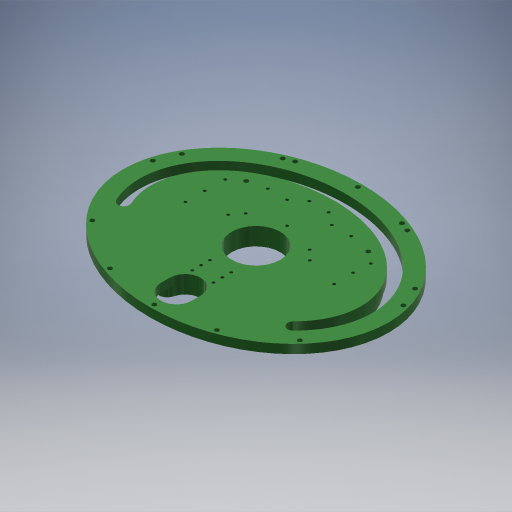
# Autodesk Inventor part: 24_0497_006
Saved by Autodesk Inventor 2024.3 (Build 283343000, 343)
## iProperties
Created: 2024-05-28
Part Number: 24_0497_006
Material: LCP-Kunststoff
Document SubType Name: Modeling
Designer: Vogel
Density: 1.626 g/cm^3
Appearance: Glatt - Waldgrün
Author: Vogel
Autodesk Inventor part; units mm, degrees
ref_plane "YZ Plane" through (0, 0, 0) normal (1, 0, 0) x (0, 1, 0)
ref_plane "XZ Plane" through (0, 0, 0) normal (0, 1, 0) x (-1, 0, 0)
ref_plane "XY Plane" through (0, 0, 0) normal (0, 0, 1) x (1, 0, 0)
sketch "Skizze1" plane through (0, 0, 0) normal (0, 0, 1) x (1, 0, 0)
  line L0 (-210, 0) -> (210, 0) projected
  line L1 (0, -168) -> (0, 168) projected
  ellipse E0 centre (0, 0) end of major axis (-150, 0) minor radius 120
  line L2 (0, 120) -> (0, -120) construction
  line L3 (-150, 0) -> (150, 0) construction
  dimension "d0" = 300
  dimension "d1" = 240
  constraints: 4 end point, 4 point on line, 1 coincident, 6 other
  measures "d0" distance of L3.start L3.end
  measures "d1" distance of L2.start L2.end
extrude "Extrusion1" add sketch "Skizze1" along normal blind 10
sketch "Skizze2" plane through (0, 0, 10) normal (0, 0, 1) x (1, 0, 0)
  ellipse E0 centre (0, 0) end of major axis (-150, 0) minor radius 120 projected
  line L0 (0, -168) -> (0, 168) projected
  line L1 (-210, 0) -> (210, 0) projected
  line L2 (-131.5, 0) -> (131.5, 0)
  line L3 (0, 101.5) -> (0, -101.5)
  ellipse E1 centre (0, 0) end of major axis (-131.5, 0) minor radius 101.5
  line L4 (0, 0) -> (-124.2275, -33.2867) construction
  line L5 (0, 0) -> (105.3012, -60.7957) construction
  ellipse E2 centre (0, 0) end of major axis (118.5, 0) minor radius 88.5
  line L6 (0, 0) -> (80.349, 80.349) construction
  line L7 (80.349, 80.349) -> (73.764, 69.2632)
  line L8 (67.3414, 73.0783) -> (84.3123, 62.9974)
  arc A0 (94.9826, -52.9176) -> (105.1165, -60.6891) centre (99.5391, -57.469) ccw
  arc A1 (-124.1391, -33.263) -> (-112.0157, -28.8739) centre (-117.8892, -31.5883) ccw
  point P0 (0, 120)
  point P1 (150, 0)
  point P2 (-150, 0)
  point P3 (0, -120)
  point P4 (118.5, 0)
  point P5 (-96, 0)
  point P6 (0, 88.5)
  point P7 (-123.7552, -34.3188)
  point P8 (104.0928, -62.0231)
  dimension "d7" = 18.5
  dimension "d8" = 18.5
  dimension "d9" = 31.5
  dimension "d10" = 31.5
  dimension "d11" = 45
  dimension "d12" = 90
  dimension "d13" = 12.8941
  dimension "d14" = 30
  dimension "d15" = 15
  constraints: 16 point on line, 14 end point, 7 coincident, 4 point on circle, 2 centre point, 2 horizontal, 2 symmetric about line, 24 other
  measures "d7" distance of point (0, 120) L3.start
  measures "d8" distance of L2.end point (150, 0)
  measures "d9" distance of point (0, 120) point (0, 88.5)
  measures "d10" distance of point (150, 0) point (118.5, 0)
  measures "d11" angle of L6 L1
  measures "d12" angle of L8 L7
  measures "d13" distance of L6.end L7.end
  measures "d14" angle of L2 L5
  measures "d15" angle of L2 L4
extrude "Extrusion2" cut sketch "Skizze2" against normal through all contours E1 L0 E2 L1 | L1 E2 A1 E1 | E1 L7 E2 L0 | E1 A0 E2 L1 | L1 E2 L7 E1
sketch "Skizze3" plane through (0, 0, 0) normal (0, 0, -1) x (-1, 0, 0)
  arc A0 (-104.0928, -62.0231) -> (-94.9826, -52.9176) centre (-99.5391, -57.469) ccw projected
  ellipse E0 centre (0, 0) end of major axis (131.5, 0) minor radius 101.5 (123.7552, -34.3188) -> (-104.0928, -62.0231) ccw projected
  arc A1 (112.0157, -28.8739) -> (123.7552, -34.3188) centre (117.8892, -31.5883) ccw projected
  ellipse E1 centre (0, 0) end of major axis (118.5, 0) minor radius 88.5 (112.0157, -28.8739) -> (-94.9826, -52.9176) ccw projected
  ellipse E2 centre (0, 0) end of major axis (150, 0) minor radius 120 projected
  line L0 (0, 0) -> (0, 120)
  line L1 (0, 0) -> (-150, 0)
  ellipse E3 centre (0, 0) end of major axis (-116, 0) minor radius 86
  circle A2 centre (0, -95.478) radius 8.75 projected
  line L2 (210, 0) -> (-210, 0) projected
  line L3 (0, -168) -> (0, 168) projected
  point P0 (0, 86)
  point P1 (-116, 0)
  point P2 (0, -86)
  point P3 (0, -86.728)
  dimension "d18" = 34
  dimension "d19" = 34
  constraints: 4 end point, 3 point on line, 2 horizontal, 1 coincident, 1 vertical, 1 vertical alignment, 11 other
  measures "d18" distance of point (-116, 0) L1.end
  measures "d19" distance of point (0, 86) L0.end
extrude "Extrusion3" add sketch "Skizze3" along normal blind 10 contours E3 L0 L1 | L1 L3 E3 | E3 L2 L0 | L2 E3 L3
sketch "Skizze4" plane through (0, 0, 10) normal (0, 0, 1) x (1, 0, 0)
  line L0 (-210, 0) -> (210, 0) projected
  line L1 (0, -168) -> (0, 168) projected
  circle A0 centre (0, -80) radius 17.5
  point P0 (0, 0)
  dimension "d22" = 35
  dimension "d23" = 80
  constraints: 1 centre point, 1 point on line
  measures "d22" diameter of A0
  measures "d23" distance from line of A0.centre L0
extrude "Extrusion4" cut sketch "Skizze4" against normal through all
sketch "Skizze5" plane through (0, 0, 10) normal (0, 0, 1) x (1, 0, 0)
  circle A0 centre (0, 0) radius 27.5
  dimension "d26" = 55
  constraints: 1 centre point, 1 coincident
  measures "d26" diameter of A0
extrude "Extrusion5" cut sketch "Skizze5" against normal through all
sketch "Skizze6" plane through (0, 0, -10) normal (0, 0, -1) x (-1, 0, 0)
  line L0 (210, 0) -> (-210, 0) projected
  line L1 (0, -168) -> (0, 168) projected
  line L2 (-12, -50) -> (-12, -40)
  line L3 (12, -50) -> (12, -40)
  line L4 (12, -50) -> (12, -60)
  line L5 (-12, -50) -> (-12, -60)
  point P0 (0, 0)
  point P1 (12, -45)
  dimension "d29" = 24
  dimension "d30" = 50
  dimension "d31" = 10
  dimension "d89" = 10
  constraints: 8 end point, 6 coincident, 4 vertical, 3 horizontal alignment, 1 midpoint, 1 other
  measures "d29" distance from line of L2 point (12, -45)
  measures "d30" distance from line of L0 L3.start
  measures "d31" distance of L3.end L3.start
  measures "d89" distance of L4.start L4.end
hole "Bohrung1" at (12, -50, -10) at (12, -40, -10) at (-12, -40, -10) at (-12, -50, -10) at (-12, -60, -10) at (12, -60, -10) direction (0, 0, 1) diameter 3.242 end through all thread size "M4x0.7" class "6H" standard "ISO Metric profile"
sketch "Skizze7" plane through (0, 0, 0) normal (0, 0, -1) x (-1, 0, 0)
  circle A0 centre (0, -115) radius 1.621 projected
  circle A1 centre (-117.2282, -67.6817) radius 1.621 projected
  circle A2 centre (117.2282, -67.6817) radius 1.621 projected
  circle A3 centre (0, 115) radius 1.621 projected
  circle A4 centre (131.7852, 47.9659) radius 1.621 projected
  circle A5 centre (70.3971, 100.5374) radius 1.621 projected
  circle A6 centre (-70.3971, 100.5374) radius 1.621 projected
  circle A7 centre (-131.7852, 47.9659) radius 1.621 projected
  arc A8 (16.8617, 59.8458) -> (2.0406, 61.4653) centre (0.7319, -19.1414) ccw projected
  arc A9 (18.3431, 57.2081) -> (16.8617, 59.8458) centre (16.4616, 57.8862) ccw projected
  line L0 (18.3431, 57.2081) -> (11.1831, 37.3438) projected
  arc A10 (8.9188, 36.0589) -> (11.1831, 37.3438) centre (9.3016, 38.0219) ccw projected
  arc A11 (8.9188, 36.0589) -> (-6.3449, 36.18) centre (0.9627, -4.7433) ccw projected
  arc A12 (-8.5965, 37.5246) -> (-6.3449, 36.18) centre (-6.6965, 38.1489) ccw projected
  line L1 (-8.5965, 37.5246) -> (-15.1484, 57.464) projected
  arc A13 (-13.6228, 60.053) -> (-15.1484, 57.464) centre (-13.2484, 58.0883) ccw projected
  arc A14 (2.0406, 61.4653) -> (-13.6228, 60.053) centre (1.3614, -18.5666) ccw projected
  line L2 (6.9792, -31.0574) -> (-7.1206, -31.0613) projected
  arc A15 (-9.1211, -29.0618) -> (-7.1206, -31.0613) centre (-7.1211, -29.0613) ccw projected
  line L3 (-9.1211, -29.0618) -> (-9.1234, -20.9579) projected
  arc A16 (-7.1239, -18.9573) -> (-9.1234, -20.9579) centre (-7.1234, -20.9573) ccw projected
  line L4 (-7.1239, -18.9573) -> (6.9759, -18.9534) projected
  arc A17 (8.9764, -20.9528) -> (6.9759, -18.9534) centre (6.9764, -20.9534) ccw projected
  line L5 (8.9764, -20.9528) -> (8.9787, -29.0568) projected
  arc A18 (6.9792, -31.0574) -> (8.9787, -29.0568) centre (6.9787, -29.0574) ccw projected
  line L6 (56.8804, 38.6385) -> (35.5944, 25.5797) projected
  arc A19 (33.209, 25.7992) -> (35.5944, 25.5797) centre (34.5485, 27.2844) ccw projected
  arc A20 (33.209, 25.7992) -> (21.3418, 32.6941) centre (10.9014, 1.0642) ccw projected
  arc A21 (20.1931, 35.5138) -> (21.3418, 32.6941) centre (21.9687, 34.5933) ccw projected
  line L7 (20.1931, 35.5138) -> (30.1934, 54.8027) projected
  arc A22 (32.5335, 55.8009) -> (30.1934, 54.8027) centre (31.9689, 53.8822) ccw projected
  arc A23 (57.1918, 41.8123) -> (32.5335, 55.8009) centre (14.9685, -3.8891) ccw projected
  arc A24 (56.8804, 38.6385) -> (57.1918, 41.8123) centre (55.8346, 40.3433) ccw projected
  line L8 (-27.611, 55.4356) -> (-18.0818, 35.9123) projected
  arc A25 (-19.301, 33.1204) -> (-18.0818, 35.9123) centre (-19.8791, 35.035) ccw projected
  arc A26 (-19.301, 33.1204) -> (-31.3271, 26.5166) centre (-9.7404, 1.4574) ccw projected
  arc A27 (-33.7193, 26.353) -> (-31.3271, 26.5166) centre (-32.6324, 28.0319) ccw projected
  line L9 (-33.7193, 26.353) -> (-54.6811, 39.9224) projected
  arc A28 (-54.9146, 43.1035) -> (-54.6811, 39.9224) centre (-53.5943, 41.6013) ccw projected
  arc A29 (-29.9275, 56.4898) -> (-54.9146, 43.1035) centre (-13.7339, -3.7518) ccw projected
  arc A30 (-27.611, 55.4356) -> (-29.9275, 56.4898) centre (-29.4083, 54.5583) ccw projected
  line L10 (-63.304, 32.0168) -> (-40.3867, 20.4807) projected
  arc A31 (-39.7038, 17.4709) -> (-40.3867, 20.4807) centre (-41.286, 18.6943) ccw projected
  arc A32 (-39.7038, 17.4709) -> (-44.03, 6.4891) centre (-22.9809, 4.54) ccw projected
  arc A33 (-46.0749, 4.6742) -> (-44.03, 6.4891) centre (-46.0214, 6.6735) ccw projected
  line L11 (-46.0749, 4.6742) -> (-73.498, 5.4071) projected
  arc A34 (-75.4382, 7.5663) -> (-73.498, 5.4071) centre (-73.4446, 7.4063) ccw projected
  arc A35 (-65.7466, 31.5025) -> (-75.4382, 7.5663) centre (-32.5314, 4.1237) ccw projected
  arc A36 (-63.304, 32.0168) -> (-65.7466, 31.5025) centre (-64.2033, 30.2304) ccw projected
  line L12 (74.722, 4.4411) -> (47.2692, 4.0773) projected
  arc A37 (45.2489, 5.9191) -> (47.2692, 4.0773) centre (47.2427, 6.0771) ccw projected
  arc A38 (45.2489, 5.9191) -> (41.0707, 16.9588) centre (24.1594, 4.2478) ccw projected
  arc A39 (41.7944, 19.9588) -> (41.0707, 16.9588) centre (42.6695, 18.1605) ccw projected
  line L13 (41.7944, 19.9588) -> (64.8807, 31.193) projected
  arc A40 (67.2895, 30.6784) -> (64.8807, 31.193) centre (65.7559, 29.3946) ccw projected
  arc A41 (76.6934, 6.5325) -> (67.2895, 30.6784) centre (36.2275, 4.6768) ccw projected
  arc A42 (74.722, 4.4411) -> (76.6934, 6.5325) centre (74.6955, 6.4409) ccw projected
  circle A43 centre (-78.9129, 21.3732) radius 1.621 projected
  circle A44 centre (-0.1326, -39.4754) radius 1.621 projected
  circle A45 centre (0.0945, -10.225) radius 1.621 projected
  circle A46 centre (-36.788, 10.5195) radius 1.621 projected
  circle A47 centre (-23, 26.9845) radius 1.621 projected
  circle A48 centre (-47.3607, 54.9329) radius 1.621 projected
  circle A49 centre (1.8344, 66.7175) radius 1.621 projected
  circle A50 centre (1.0847, 32.3926) radius 1.621 projected
  circle A51 centre (23.7748, 26.5486) radius 1.621 projected
  circle A52 centre (38.2131, 10.8708) radius 1.621 projected
  circle A53 centre (49.4396, 53.9051) radius 1.621 projected
  circle A54 centre (80.7711, 19.9099) radius 1.621 projected
  ellipse E0 centre (0, 0) end of major axis (150, 0) minor radius 120 projected
  arc A55 (-126.5358, -22.9315) -> (-116.9938, -20.0189) centre (-121.7662, -21.4707) ccw projected
  ellipse E1 centre (0, 0) end of major axis (130, 0) minor radius 100 (122.4016, -33.6872) -> (-126.5358, -22.9315) ccw projected
  arc A56 (113.3712, -29.4986) -> (122.4016, -33.6872) centre (117.8886, -31.5882) ccw projected
  ellipse E2 centre (0, 0) end of major axis (120, 0) minor radius 90 (113.3712, -29.4986) -> (-116.9938, -20.0189) ccw projected
  constraints: 8 coincident, 2 other
hole "Bohrung2" at (-131.7852, 47.9659, 0) at (-70.3971, 100.5374, 0) at (-117.2282, -67.6817, 0) at (0, -115, 0) at (117.2282, -67.6817, 0) at (131.7852, 47.9659, 0) at (70.3971, 100.5374, 0) at (0, 115, 0) direction (0, 0, 1) diameter 5.2 end through all
sketch "Skizze9" plane through (0, 0, 0) normal (0, 0, -1) x (-1, 0, 0)
  circle A0 centre (0, 115) radius 2.6 projected
  circle A1 centre (-70.3971, 100.5374) radius 2.6 projected
  circle A2 centre (-131.7852, 47.9659) radius 2.6 projected
  circle A3 centre (-117.2282, -67.6817) radius 2.6 projected
  circle A4 centre (0, -115) radius 2.6 projected
  circle A5 centre (117.2282, -67.6817) radius 2.6 projected
  circle A6 centre (70.3971, 100.5374) radius 2.6 projected
  circle A7 centre (131.7852, 47.9659) radius 2.6 projected
  ellipse E0 centre (0, 0) end of major axis (150, 0) minor radius 120 projected
  arc A8 (-104.0928, -62.0231) -> (-94.9826, -52.9176) centre (-99.5391, -57.469) ccw projected
  ellipse E1 centre (0, 0) end of major axis (131.5, 0) minor radius 101.5 (123.7552, -34.3188) -> (-104.0928, -62.0231) ccw projected
  arc A9 (112.0157, -28.8739) -> (123.7552, -34.3188) centre (117.8892, -31.5883) ccw projected
  ellipse E2 centre (0, 0) end of major axis (118.5, 0) minor radius 88.5 (112.0157, -28.8739) -> (-94.9826, -52.9176) ccw projected
  arc A10 (-16.7404, -85.0997) -> (16.7404, -85.0997) centre (0, -80) ccw projected
  ellipse E3 centre (0, 0) end of major axis (-116, 0) minor radius 86 (16.7404, -85.0997) -> (-16.7404, -85.0997) ccw projected
  line L0 (0, -168) -> (0, 168) construction
  line L1 (210, 0) -> (-210, 0) projected
  line L2 (0, 0) -> (-145, 0) construction
  line L3 (0, 0) -> (0, 115)
  ellipse E4 centre (0, 0) end of major axis (-145, 0) minor radius 115 construction
  line L4 (0, 0) -> (-60.3676, 104.5597)
  line L5 (0, 0) -> (60.3676, 104.5597)
  line L6 (0, 0) -> (-141.544, 24.958)
  line L7 (0, 0) -> (141.544, 24.958)
  line L8 (0, 0) -> (-60.3676, -104.5597)
  line L9 (0, 0) -> (60.3676, -104.5597)
  dimension "d46" = 145
  dimension "d47" = 30
  dimension "d48" = 10
  constraints: 16 end point, 7 coincident, 2 collinear, 1 horizontal, 1 perpendicular, 1 point on line, 15 other
  measures "d46" distance of L2.end point (0, 0)
  measures "d47" angle of L4 L3
  measures "d48" angle of L6 L1
hole "Bohrung3" at (141.544, 24.958, 0) at (60.3676, 104.5597, 0) at (-60.3676, 104.5597, 0) at (-141.544, 24.958, 0) at (60.3676, -104.5597, 0) at (-60.3676, -104.5597, 0) direction (0, 0, 1) diameter 5.2 end through all
sketch "Skizze10" plane through (0, 0, 10) normal (0, 0, 1) x (1, 0, 0)
  circle A0 centre (44.6817, 16.1402) radius 2.2 projected
  circle A1 centre (34.1537, 26.537) radius 2.2 projected
  circle A2 centre (81.1696, 28.4843) radius 2.2 projected
  circle A3 centre (81.5761, 6.6779) radius 2.1999 projected
  circle A4 centre (44.3119, 63.2458) radius 2.2 projected
  circle A5 centre (22.5018, 63.252) radius 2.1999 projected
  circle A6 centre (8.2159, 73.8332) radius 2.2001 projected
  circle A7 centre (-13.5942, 73.8394) radius 2.2 projected
  circle A8 centre (-1.9423, 37.1245) radius 2.2 projected
  circle A9 centre (-37.5824, 25.8885) radius 2.2 projected
  circle A10 centre (-46.0331, 14.7062) radius 2.2 projected
  circle A11 centre (-60.3676, -104.5597) radius 2.6 projected
  circle A12 centre (60.3676, -104.5597) radius 2.6 projected
  circle A13 centre (-141.544, 24.958) radius 2.6 projected
  circle A14 centre (-60.3676, 104.5597) radius 2.6 projected
  circle A15 centre (60.3676, 104.5597) radius 2.6 projected
  circle A16 centre (141.544, 24.958) radius 2.6 projected
  circle A17 centre (0, 115) radius 2.6 projected
  circle A18 centre (70.3971, 100.5374) radius 2.6 projected
  circle A19 centre (131.7852, 47.9659) radius 2.6 projected
  circle A20 centre (117.2282, -67.6817) radius 2.6 projected
  circle A21 centre (0, -115) radius 2.6 projected
  circle A22 centre (-117.2282, -67.6817) radius 2.6 projected
  circle A23 centre (-70.3971, 100.5374) radius 2.6 projected
  circle A24 centre (-131.7852, 47.9659) radius 2.6 projected
  circle A25 centre (-12, -50) radius 1.621 projected
  circle A26 centre (-12, -40) radius 1.621 projected
  circle A27 centre (12, -40) radius 1.621 projected
  circle A28 centre (12, -50) radius 1.621 projected
  circle A29 centre (0, 0) radius 27.5 projected
  circle A30 centre (0, -80) radius 17.5 projected
  arc A31 (94.9826, -52.9176) -> (104.0928, -62.0231) centre (99.5391, -57.469) ccw projected
  ellipse E0 centre (0, 0) end of major axis (-118.5, 0) minor radius 88.5 (94.9826, -52.9176) -> (-112.0157, -28.8739) ccw projected
  arc A32 (-123.7552, -34.3188) -> (-112.0157, -28.8739) centre (-117.8892, -31.5883) ccw projected
  ellipse E1 centre (0, 0) end of major axis (-131.5, 0) minor radius 101.5 (104.0928, -62.0231) -> (-123.7552, -34.3188) ccw projected
  ellipse E2 centre (0, 0) end of major axis (-150, 0) minor radius 120 projected
  circle A33 centre (-82.748, 3.0543) radius 2.2 projected
  circle A34 centre (-82.7416, 24.8646) radius 2.2003 projected
  circle A35 centre (-49.2342, 62.6034) radius 2.2001 projected
  circle A36 centre (-27.4241, 62.5973) radius 2.2 projected
  constraints: 15 coincident, 3 other
hole "Bohrung4" at (81.1696, 28.4843, 10) at (81.5761, 6.6779, 10) at (44.6817, 16.1402, 10) at (34.1537, 26.537, 10) at (44.3119, 63.2458, 10) at (22.5018, 63.252, 10) at (-13.5942, 73.8394, 10) at (-1.9423, 37.1245, 10) at (8.2159, 73.8332, 10) at (-27.4241, 62.5973, 10) at (-37.5824, 25.8885, 10) at (-46.0331, 14.7062, 10) at (-49.2342, 62.6034, 10) at (-82.7416, 24.8646, 10) at (-82.748, 3.0543, 10) direction (0, 0, -1) diameter 3.242 end through all thread size "M4x0.7" class "6H" standard "ISO Metric profile"
sketch "Skizze11" plane through (0, 0, -10) normal (0, 0, -1) x (-1, 0, 0)
  circle A0 centre (82.748, 3.0543) radius 1.621 projected
  circle A1 centre (82.7416, 24.8646) radius 1.621 projected
  circle A2 centre (49.2342, 62.6034) radius 1.621 projected
  circle A3 centre (46.0331, 14.7062) radius 1.621 projected
  circle A4 centre (37.5824, 25.8885) radius 1.621 projected
  circle A5 centre (27.4241, 62.5973) radius 1.621 projected
  circle A6 centre (-8.2159, 73.8332) radius 1.621 projected
  circle A7 centre (1.9423, 37.1245) radius 1.621 projected
  circle A8 centre (13.5942, 73.8394) radius 1.621 projected
  circle A9 centre (-22.5018, 63.252) radius 1.621 projected
  circle A10 centre (-44.3119, 63.2458) radius 1.621 projected
  circle A11 centre (-34.1537, 26.537) radius 1.621 projected
  circle A12 centre (-44.6817, 16.1402) radius 1.621 projected
  circle A13 centre (-81.5761, 6.6779) radius 1.621 projected
  circle A14 centre (-81.1696, 28.4843) radius 1.621 projected
  circle A15 centre (12, -50) radius 1.621 projected
  circle A16 centre (12, -40) radius 1.621 projected
  circle A17 centre (-12, -40) radius 1.621 projected
  circle A18 centre (-12, -50) radius 1.621 projected
  circle A19 centre (0, 0) radius 27.5 projected
  arc A20 (16.7404, -85.0997) -> (-16.7404, -85.0997) centre (0, -80) ccw projected
  ellipse E0 centre (0, 0) end of major axis (-116, 0) minor radius 86 (16.7404, -85.0997) -> (-16.7404, -85.0997) ccw projected
  line L0 (0, 0) -> (-91.5217, 52.8401)
  line L1 (0, 0) -> (91.5217, 52.8401)
  line L2 (210, 0) -> (-210, 0) projected
  line L3 (0, -168) -> (0, 168) projected
  point P0 (82.2724, 47.5)
  point P1 (-82.2724, 47.5)
  dimension "d63" = 60
  dimension "d64" = 60
  dimension "d65" = 95
  dimension "d66" = 95
  constraints: 4 end point, 2 point on line, 3 other
  measures "d63" angle of L1 L3
  measures "d64" angle of L3 L0
  measures "d65" distance of point (-82.272, 47.5) point (0, 0)
  measures "d66" distance of point (82.272, 47.5) point (0, 0)
hole "Bohrung5" at (-82.2724, 47.5, -10) at (82.2724, 47.5, -10) direction (0, 0, 1) diameter 3.242 end through all thread size "M4x0.7" class "6H" standard "ISO Metric profile"
sketch "Skizze13" plane through (0, 0, -10) normal (0, 0, -1) x (-1, 0, 0)
  circle A0 centre (-82.2724, 47.5) radius 1.621 projected
  circle A1 centre (82.2724, 47.5) radius 1.621 projected
  circle A2 centre (82.748, 3.0543) radius 1.621 projected
  circle A3 centre (82.7416, 24.8646) radius 1.621 projected
  circle A4 centre (49.2342, 62.6034) radius 1.621 projected
  circle A5 centre (46.0331, 14.7062) radius 1.621 projected
  circle A6 centre (37.5824, 25.8885) radius 1.621 projected
  circle A7 centre (27.4241, 62.5973) radius 1.621 projected
  circle A8 centre (-8.2159, 73.8332) radius 1.621 projected
  circle A9 centre (1.9423, 37.1245) radius 1.621 projected
  circle A10 centre (13.5942, 73.8394) radius 1.621 projected
  circle A11 centre (-22.5018, 63.252) radius 1.621 projected
  circle A12 centre (-44.3119, 63.2458) radius 1.621 projected
  circle A13 centre (-34.1537, 26.537) radius 1.621 projected
  circle A14 centre (-44.6817, 16.1402) radius 1.621 projected
  circle A15 centre (-81.5761, 6.6779) radius 1.621 projected
  circle A16 centre (-81.1696, 28.4843) radius 1.621 projected
  circle A17 centre (12, -50) radius 1.621 projected
  circle A18 centre (12, -40) radius 1.621 projected
  circle A19 centre (-12, -40) radius 1.621 projected
  circle A20 centre (-12, -50) radius 1.621 projected
  circle A21 centre (0, 0) radius 27.5 projected
  arc A22 (16.7404, -85.0997) -> (-16.7404, -85.0997) centre (0, -80) ccw projected
  ellipse E0 centre (0, 0) end of major axis (-116, 0) minor radius 86 (16.7404, -85.0997) -> (-16.7404, -85.0997) ccw projected
  circle A23 centre (60.3676, 104.5597) radius 2.6 projected
  circle A24 centre (-60.3676, 104.5597) radius 2.6 projected
  line L0 (210, 0) -> (-210, 0) projected
  line L1 (0, -168) -> (0, 168) projected
  line L2 (0, 0) -> (76.8062, 64.448)
  line L3 (0, 0) -> (-76.8062, 64.448)
  point P0 (68.944, 57.8509)
  point P1 (-68.944, 57.8509)
  dimension "d74" = 50
  dimension "d75" = 50
  dimension "d76" = 90
  dimension "d77" = 90
  constraints: 4 end point, 2 point on line, 3 other
  measures "d74" angle of L1 L2
  measures "d75" angle of L3 L1
  measures "d76" distance of point (0, 0) point (68.944, 57.851)
  measures "d77" distance of point (0, 0) point (-68.944, 57.851)
hole "Bohrung6" at (-68.944, 57.8509, -10) at (68.944, 57.8509, -10) direction (0, 0, 1) diameter 5.2 end through all
sketch "Skizze14" plane through (0, 0, 10) normal (0, 0, 1) x (1, 0, 0)
  ellipse E0 centre (0, 0) end of major axis (116, 0) minor radius 86 (16.7404, -85.0997) -> (-16.7404, -85.0997) ccw projected
  circle A0 centre (68.944, 57.8509) radius 2.6 projected
  circle A1 centre (-68.944, 57.8509) radius 2.6 projected
  circle A2 centre (82.2724, 47.5) radius 1.621 projected
  circle A3 centre (-82.2724, 47.5) radius 1.621 projected
  circle A4 centre (-82.748, 3.0543) radius 1.621 projected
  circle A5 centre (-82.7416, 24.8646) radius 1.621 projected
  circle A6 centre (-49.2342, 62.6034) radius 1.621 projected
  circle A7 centre (-46.0331, 14.7062) radius 1.621 projected
  circle A8 centre (-37.5824, 25.8885) radius 1.621 projected
  circle A9 centre (-27.4241, 62.5973) radius 1.621 projected
  circle A10 centre (8.2159, 73.8332) radius 1.621 projected
  circle A11 centre (-1.9423, 37.1245) radius 1.621 projected
  circle A12 centre (-13.5942, 73.8394) radius 1.621 projected
  circle A13 centre (22.5018, 63.252) radius 1.621 projected
  circle A14 centre (44.3119, 63.2458) radius 1.621 projected
  circle A15 centre (34.1537, 26.537) radius 1.621 projected
  circle A16 centre (44.6817, 16.1402) radius 1.621 projected
  circle A17 centre (81.5761, 6.6779) radius 1.621 projected
  circle A18 centre (81.1696, 28.4843) radius 1.621 projected
  circle A19 centre (-60.3676, -104.5597) radius 2.6 projected
  circle A20 centre (60.3676, -104.5597) radius 2.6 projected
  circle A21 centre (-141.544, 24.958) radius 2.6 projected
  circle A22 centre (-60.3676, 104.5597) radius 2.6 projected
  circle A23 centre (60.3676, 104.5597) radius 2.6 projected
  circle A24 centre (141.544, 24.958) radius 2.6 projected
  circle A25 centre (0, 115) radius 2.6 projected
  circle A26 centre (70.3971, 100.5374) radius 2.6 projected
  circle A27 centre (131.7852, 47.9659) radius 2.6 projected
  circle A28 centre (117.2282, -67.6817) radius 2.6 projected
  circle A29 centre (0, -115) radius 2.6 projected
  circle A30 centre (-117.2282, -67.6817) radius 2.6 projected
  circle A31 centre (-70.3971, 100.5374) radius 2.6 projected
  circle A32 centre (-131.7852, 47.9659) radius 2.6 projected
  circle A33 centre (-12, -50) radius 1.621 projected
  circle A34 centre (-12, -40) radius 1.621 projected
  circle A35 centre (12, -40) radius 1.621 projected
  circle A36 centre (12, -50) radius 1.621 projected
  circle A37 centre (0, 0) radius 27.5 projected
  circle A38 centre (0, -80) radius 17.5 projected
  arc A39 (94.9826, -52.9176) -> (104.0928, -62.0231) centre (99.5391, -57.469) ccw projected
  ellipse E1 centre (0, 0) end of major axis (-118.5, 0) minor radius 88.5 (94.9826, -52.9176) -> (-112.0157, -28.8739) ccw projected
  arc A40 (-123.7552, -34.3188) -> (-112.0157, -28.8739) centre (-117.8892, -31.5883) ccw projected
  ellipse E2 centre (0, 0) end of major axis (-131.5, 0) minor radius 101.5 (104.0928, -62.0231) -> (-123.7552, -34.3188) ccw projected
  ellipse E3 centre (0, 0) end of major axis (-150, 0) minor radius 120 projected
  line L0 (-210, 0) -> (210, 0) projected
  line L1 (0, -168) -> (0, 168) projected
  line L2 (0, -80) -> (0, -90) construction
  line L3 (-17.5, -80) -> (-17.5, -90)
  line L4 (17.5, -90) -> (17.5, -80)
  arc A41 (17.5, -80) -> (-17.5, -80) centre (0, -80) ccw
  arc A42 (-17.5, -90) -> (17.5, -90) centre (0, -90) ccw
  point P0 (0, -85)
  point P1 (17.5, -85.0157)
  point P2 (16.7404, -85.0997)
  point P3 (-16.7404, -85.0997)
  point P4 (-17.5, -85.0157)
  dimension "d85" = 10
  constraints: 8 end point, 5 tangent, 4 point on circle, 2 centre point, 1 midpoint, 1 parallel, 1 point on line, 4 other
  measures "d85" distance of L4.start L4.end
extrude "Extrusion6" cut sketch "Skizze14" against normal through all contours A38 L4 E0 | A38 L1 | E0 L4 A42 L1 A38 | L1 A42 L3 E0 A38 | A38 L1 | E0 L3 A38
fillet "Rundung1" radius 10 2 edges at (-17.5, -85.0157, -5) (17.5, -85.0157, -5)
sketch "Skizze15" plane through (0, 0, 10) normal (0, 0, 1) x (1, 0, 0)
  ellipse E0 centre (0, 0) end of major axis (116, 0) minor radius 86 (28.5782, -83.3493) -> (-28.5782, -83.3493) ccw projected
  circle A0 centre (0, -88.2147) radius 2.5 projected
  arc A1 (17.5, -80) -> (-17.5, -80) centre (0, -80) ccw projected
  circle A2 centre (0, -88.2147) radius 11.5 projected
  line L0 (-210, 0) -> (210, 0) projected
  line L1 (0, -168) -> (0, 168) projected
  point P0 (0, -62.5)
  point P1 (0, -76.7147)
  dimension "d91" = 23
  dimension "d90" = 25.7147
  constraints: 1 point on circle, 1 point on line, 1 vertical alignment, 2 other
  measures "d90" distance of point (0, -62.5) A0.centre
equation "\"d8\" = d7"
equation "\"d10\" = d9"
equation "\"d19\" = d18"
equation "\"d63\" = d64"
equation "\"d66\" = d65"
equation "\"d74\" = d75"
equation "\"d76\" = d77"
